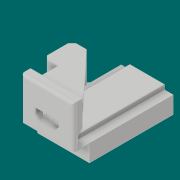
# Autodesk Inventor part: pro_micro_mount
Saved by Autodesk Inventor 2019 (Build 230136000, 136)
## iProperties
Created: 2021-04-17
Part Number: pro_micro_mount
Material: Generic
Document SubType Name: Modeling
Designer: Jacob
Density: 1 g/cm^3
Appearance: Default
Author: Jacob
Autodesk Inventor part; units mm, degrees
ref_plane "YZ Plane" through (0, 0, 0) normal (1, 0, 0) x (0, 1, 0)
ref_plane "XZ Plane" through (0, 0, 0) normal (0, 1, 0) x (-1, 0, 0)
ref_plane "XY Plane" through (0, 0, 0) normal (0, 0, 1) x (1, 0, 0)
sketch "Sketch1" plane through (0, 0, 0) normal (1, 0, 0) x (0, 1, 0)
  line L0 (0, 0) -> (5.55, 0)
  line L1 (5.55, 0) -> (5.55, 5.6)
  line L2 (5.55, 5.6) -> (20.55, 5.6)
  line L3 (20.55, 5.6) -> (20.55, 2.4)
  line L4 (20.55, 2.4) -> (10.05, 2.4)
  line L5 (10.05, 2.4) -> (10.05, 4)
  line L6 (10.05, 4) -> (7.55, 4)
  line L7 (7.55, 4) -> (7.55, -29)
  line L8 (0, 0) -> (0, -29)
  line L9 (0, -29) -> (7.55, -29)
  dimension "d1" = 5.55
  dimension "d2" = 15
  dimension "d3" = 2
  dimension "d4" = 2.5
  dimension "d5" = 1.6
  dimension "d6" = 29
  dimension "d7" = 33
  dimension "d8" = 3.2
  constraints: 20 end point, 8 perpendicular, 1 horizontal, 1 vertical
  measures "d1" distance of L0.start L0.end
  measures "d2" distance of L1.end L2.end
  measures "d3" distance between parallel lines of L1 L7
  measures "d4" distance between parallel lines of L5 L7
  measures "d5" distance between parallel lines of L2 L6
  measures "d6" distance of L0.start L8.end
  measures "d7" distance of L6.end L7.end
  measures "d8" distance of L2.end L3.end
extrude "Extrusion1" add sketch "Sketch1" along normal blind 18
sketch "Sketch2" plane through (0, 10.05, 2.4) normal (0, 0, -1) x (-1, 0, 0)
  line L0 (0, 0) -> (-18, 0) projected
  line L1 (-9, 0) -> (-9, -5.1044) construction
  line L2 (-13, 2.82) -> (-5, 2.82)
  line L3 (-5, 2.82) -> (-5, -0.28)
  line L4 (-5, -0.28) -> (-13, -0.28)
  line L5 (-13, -0.28) -> (-13, 2.82)
  point P0 (0, -10.05)
  point P1 (-9, -0.28)
  dimension "d11" = 3.1
  dimension "d12" = 8
  constraints: 10 end point, 2 midpoint, 2 parallel, 1 horizontal, 1 perpendicular, 1 point on line, 1 vertical
  measures "d11" distance of L2.end L3.end
  measures "d12" distance of L2.start L2.end
extrude "Extrusion2" cut sketch "Sketch2" against normal up to surface (3.2 mm away)
chamfer "Chamfer1" distance 1.2 angle 45 2 edges at (5, 9.77, 4.8) (13, 9.77, 4.8)
chamfer "Chamfer2" distance 1.6 angle 45 2 edges at (15.04, 10.05, 2.4) (2.96, 10.05, 2.4)
fillet "Fillet1" radius 1 4 edges at (9, 5.55, 5.6) (9, 20.55, 5.6) (18, 13.05, 5.6) (0, 13.05, 5.6)
sketch "Sketch3" plane through (0, 0, -29) normal (0, 0, -1) x (-1, 0, 0)
  line L0 (0, 7.55) -> (-18, 7.55) projected
  line L1 (-9, 7.55) -> (-9, 5.1292) construction
  line L2 (-18, 7.55) -> (-15, 7.55)
  line L3 (-15, 7.55) -> (-15, 5.95)
  line L4 (-15, 5.95) -> (-18, 5.95)
  line L5 (-18, 5.95) -> (-18, 7.55)
  line L6 (0, 7.55) -> (-3, 7.55)
  line L7 (-3, 7.55) -> (-3, 5.95)
  line L8 (-3, 5.95) -> (0, 5.95)
  line L9 (0, 5.95) -> (0, 7.55)
  line L10 (0, 7.55) -> (-18, 7.55) projected
  line L11 (-18, 0) -> (-18, 7.55) projected
  point P0 (0, 0)
  dimension "d22" = 3
  dimension "d23" = 1.6
  constraints: 18 end point, 4 symmetric about line, 2 collinear, 2 parallel, 1 horizontal, 1 midpoint, 1 perpendicular, 1 vertical
  measures "d22" distance of L2.start L2.end
  measures "d23" distance of L2.end L3.end
extrude "Extrusion3" cut sketch "Sketch3" against normal up to surface (33 mm away)
chamfer "Chamfer3" distance 1.6 angle 45 2 edges at (16.5, 5.95, 4) (1.5, 5.95, 4)
sketch "Sketch4" plane through (0, 0, 0) normal (-1, 0, 0) x (0, 0, 1)
  line L0 (-17, 0) -> (-7, 0)
  line L1 (-7, 0) -> (-7, 16.55)
  line L2 (-7, 16.55) -> (-17, 16.55)
  line L3 (-17, 16.55) -> (-17, 0)
  line L4 (2.4, 5.95) -> (-29, 5.95) projected
  line L5 (-29, 0) -> (0, 0) projected
  line L6 (0, 0) -> (0, 5.55) projected
  line L7 (4.6, 20.55) -> (2.4, 20.55) projected
  dimension "d29" = 10
  dimension "d30" = 7
  dimension "d31" = 4
  constraints: 8 end point, 2 parallel, 1 collinear, 1 horizontal, 1 perpendicular
  measures "d29" distance between parallel lines of L1 L3
  measures "d30" distance between parallel lines of L6 L1
  measures "d31" distance between parallel lines of L7 L2
extrude "Extrusion4" add sketch "Sketch4" along normal blind 5
sketch "Sketch5" plane through (0, 16.55, -7) normal (0, 1, 0) x (1, 0, 0)
  line L0 (0, -9.4) -> (18, -9.4) projected
  line L1 (0, 0) -> (-5, 0) projected
  line L2 (0, 0) -> (0, 10) projected
  line L3 (0, 10) -> (-5, 10) projected
  line L4 (-5, 0) -> (-5, 10) projected
  line L5 (0, 10) -> (0, 22) projected
  line L6 (-5, 10) -> (-5, 0) projected
  line L7 (0, 10) -> (-5, 10)
  line L8 (-5, 10) -> (-5, 0)
  line L9 (-5, 0) -> (0, 0)
  line L10 (13, -9.4) -> (5, -9.4) projected
  line L11 (13, -9.4) -> (18, -9.4) projected
  line L12 (5, -9.4) -> (18, -9.4)
  line L13 (18, -9.4) -> (0, 10)
  line L14 (3, -9.4) -> (0, -9.4) projected
  line L15 (0, 0) -> (0, -9.4)
  line L16 (0, -9.4) -> (18, -9.4)
  point P0 (0, -7)
  constraints: 14 end point, 3 collinear, 2 perpendicular, 1 vertical
extrude "Extrusion5" add sketch "Sketch5" against normal blind 2.5
chamfer "Chamfer4" distance 1.35 angle 45 3 edges at (-5, 8.275, -7) (-5, 8.275, -17) (0, 2.975, -17)
body "Solid1"
